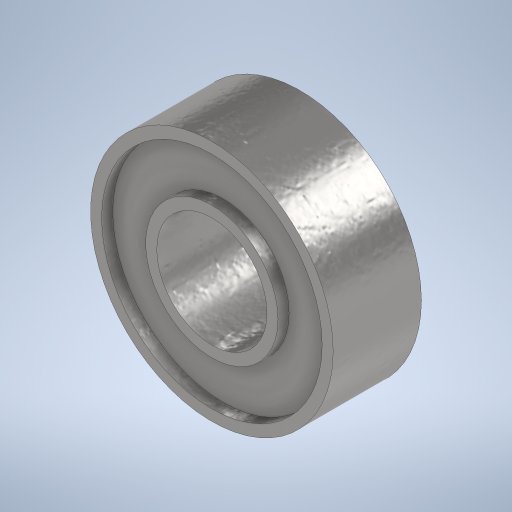
# Autodesk Inventor part: bearing 1
Saved by Autodesk Inventor 2023 (Build 270158000, 158)
## iProperties
Created: 2022-11-29
Part Number: bearing 1
Material: Steel, Galvanized
Document SubType Name: Modeling
Designer: robocin
Density: 7.85 g/cm^3
Appearance: Galvanized
Mass: 1.97292 g
Surface Area: 4.02124 cm^2
Volume: 0.251327 cm^3
Author: robocin
Autodesk Inventor part; units mm, degrees
ref_plane "YZ Plane" through (0, 0, 0) normal (1, 0, 0) x (0, 1, 0)
ref_plane "XZ Plane" through (0, 0, 0) normal (0, 1, 0) x (-1, 0, 0)
ref_plane "XY Plane" through (0, 0, 0) normal (0, 0, 1) x (1, 0, 0)
sketch "Sketch1" plane through (0, 0, 0) normal (0, 0, 1) x (1, 0, 0)
  circle A0 centre (0, 0) radius 5.5
  circle A1 centre (0, 0) radius 2.5
  dimension "d0" = 11
  dimension "d1" = 5
  constraints: 2 centre point, 2 coincident
  measures "d0" diameter of A0
  measures "d1" diameter of A1
extrude "Extrusion1" add sketch "Sketch1" along normal blind 4
sketch "Sketch2" plane through (0, 0, 4) normal (0, 0, 1) x (1, 0, 0)
  circle A0 centre (0, 0) radius 3
  circle A1 centre (0, 0) radius 5
  circle A2 centre (0, 0) radius 5.5 projected
  circle A3 centre (0, 0) radius 2.5 projected
  dimension "d4" = 0.5
  dimension "d5" = 0.5
  constraints: 2 centre point, 2 coincident
  measures "d4" radial gap between concentric circles of A2 A1
  measures "d5" radial gap between concentric circles of A3 A0
extrude "Extrusion2" cut sketch "Sketch2" against normal blind 0.5 contours A1
sketch "Sketch4" plane through (0, 0, 0) normal (0, 0, -1) x (-1, 0, 0)
  circle A0 centre (0, 0) radius 3
  circle A1 centre (0, 0) radius 5
  constraints: 2 centre point, 2 coincident
extrude "Extrusion3" cut sketch "Sketch4" against normal blind 0.5
body "Solid1"
